flaskholder100ml_v4 (Autodesk Fusion 360 design; units mm, degrees)
Autodesk Fusion 360 part; units mm, degrees
sketch "Sketch1" plane through (0, 0, 0) normal (0, 0, 1) x (1, 0, 0)
  line L0 (99, 4.8) -> (99, -4.8)
  line L1 (-99, -4.8) -> (-99, 4.8)
  line L2 (-99, 9) -> (99, -9) construction
  line L3 (99, 9) -> (-99, -9) construction
  line L4 (6, 99) -> (-4.8, 99)
  line L5 (-4.8, -99) -> (4.8, -99)
  line L6 (9, 99) -> (-9, -99) construction
  line L7 (-9, 99) -> (9, -99) construction
  line L8 (-29, -9) -> (-94.8, -9)
  line L9 (94.8, -9) -> (29, -9)
  line L10 (0.8182, -9) -> (-0.8182, -9)
  line L11 (29, 9) -> (94.8, 9)
  line L12 (-94.8, 9) -> (-31.5, 9)
  line L13 (-0.8182, 9) -> (0.8182, 9)
  line L14 (-9, 94.8) -> (-9, 31.5)
  line L15 (-9, 0.8182) -> (-9, -0.8182)
  line L16 (-9, -29) -> (-9, -94.8)
  line L17 (9, -94.8) -> (9, -29)
  line L18 (9, 29) -> (9, 96)
  arc A0 (9, 29) -> (29, 9) centre (29, 29) ccw
  arc A1 (29, -9) -> (9, -29) centre (29, -29) ccw
  arc A2 (-9, -29) -> (-29, -9) centre (-29, -29) ccw
  arc A3 (-31.5, 9) -> (-9, 31.5) centre (-31.5, 31.5) ccw
  arc A4 (9, 96) -> (6, 99) centre (6, 96) ccw
  arc A5 (-4.8, 99) -> (-9, 94.8) centre (-4.8, 94.8) ccw
  arc A6 (-94.8, 9) -> (-99, 4.8) centre (-94.8, 4.8) ccw
  arc A7 (-99, -4.8) -> (-94.8, -9) centre (-94.8, -4.8) ccw
  arc A8 (99, 4.8) -> (94.8, 9) centre (94.8, 4.8) ccw
  arc A9 (94.8, -9) -> (99, -4.8) centre (94.8, -4.8) ccw
  arc A10 (-9, -94.8) -> (-4.8, -99) centre (-4.8, -94.8) ccw
  arc A11 (4.8, -99) -> (9, -94.8) centre (4.8, -94.8) ccw
  circle A12 centre (-86, 0) radius 1
  circle A13 centre (-31, 0) radius 1
  circle A14 centre (86, 0) radius 1
  circle A15 centre (31, 0) radius 1
  circle A16 centre (0, -86) radius 1
  circle A17 centre (0, -31) radius 1
  circle A18 centre (0, 86) radius 1
  circle A19 centre (0, 31) radius 1
  circle A20 centre (0, 0) radius 1
  dimension "d1" = 198
  dimension "d2" = 18
  dimension "d5" = 18
  dimension "d6" = 198
  dimension "d9" = 20
  dimension "d10" = 22.5
  dimension "d11" = 3
  dimension "d12" = 4.2
  dimension "d15" = 2
  dimension "d16" = 2
  dimension "d17" = 13
  dimension "d18" = 2
  dimension "d19" = 13
  dimension "d20" = 2
  dimension "d21" = 2
  dimension "d22" = 13
  dimension "d23" = 2
  dimension "d24" = 2
  dimension "d25" = 13
  dimension "d26" = 68
  dimension "d27" = 68
  dimension "d28" = 68
  dimension "d29" = 68
  dimension "d30" = 2
  constraint horizontal L12
  constraint perpendicular L0 L12
  constraint parallel L9 L12
  constraint parallel L0 L1
  constraint coincident L2 A20.centre
  constraint coincident L3 A20.centre
  constraint coincident A20.centre origin
  constraint horizontal L4
  constraint perpendicular L4 L14
  constraint parallel L4 L5
  constraint parallel L14 L17
  constraint coincident L6 A20.centre
  constraint coincident L7 A20.centre
  constraint coincident L6 L10.end
  constraint collinear L8 L9
  constraint coincident L7 L10.start
  constraint collinear L9 L10
  constraint coincident L6 L13.end
  constraint collinear L11 L12
  constraint coincident L7 L13.start
  constraint collinear L12 L13
  constraint coincident L2 L15.start
  constraint collinear L14 L15
  constraint coincident L3 L15.end
  constraint collinear L15 L16
  constraint collinear L17 L18
  constraint tangent L18 A0
  constraint tangent L11 A0
  constraint tangent L9 A1
  constraint tangent L17 A1
  constraint equal A0 A1
  constraint tangent L16 A2
  constraint tangent L8 A2
  constraint equal A0 A2
  constraint tangent L12 A3
  constraint tangent L14 A3
  constraint coincident L6.start L4
  constraint coincident L6.start L18
  constraint tangent L4 A4
  constraint tangent L18 A4
  constraint coincident L7.start L4
  constraint coincident L7.start L14
  constraint tangent L4 A5
  constraint tangent L14 A5
  constraint coincident L2.start L12
  constraint coincident L2.start L1
  constraint tangent L12 A6
  constraint tangent L1 A6
  constraint equal A5 A6
  constraint coincident L3.end L1
  constraint coincident L3.end L8
  constraint tangent L1 A7
  constraint tangent L8 A7
  constraint equal A5 A7
  constraint coincident L3.start L11
  constraint coincident L3.start L0
  constraint tangent L11 A8
  constraint tangent L0 A8
  constraint equal A5 A8
  constraint coincident L2.end L9
  constraint coincident L2.end L0
  constraint tangent L9 A9
  constraint tangent L0 A9
  constraint equal A5 A9
  constraint coincident L6.end L5
  constraint coincident L6.end L16
  constraint tangent L5 A10
  constraint tangent L16 A10
  constraint equal A5 A10
  constraint coincident L7.end L17
  constraint coincident L7.end L5
  constraint tangent L17 A11
  constraint tangent L5 A11
  constraint equal A5 A11
  constraint equal A12 A14
  measures "d1" distance of L2.end L3.end
  measures "d2" distance of L3.start L2.end
  measures "d5" distance of L6.end L7.end
  measures "d6" distance of L7.start L6.end
  measures "d9" radius of A0
  measures "d10" radius of A3
  measures "d11" radius of A4
  measures "d12" radius of A5
  measures "d15" diameter of A12
  measures "d16" diameter of A13
  measures "d17" distance of L1 A12.centre
  measures "d18" diameter of A15
  measures "d19" distance of L0 A14.centre
  measures "d20" diameter of A16
  measures "d21" diameter of A17
  measures "d22" distance of L5 A16.centre
  measures "d23" diameter of A18
  measures "d24" diameter of A19
  measures "d25" distance of L4 A18.centre
  measures "d26" distance of L4 A19.centre
  measures "d27" distance of L0 A15.centre
  measures "d28" distance of L1 A13.centre
  measures "d29" distance of L5 A17.centre
  measures "d30" diameter of A20
extrude "Extrude1" add sketch "Sketch1" along normal blind 3.175
equation "d1 = totalArmLenght"
equation "d2 = armWidth"
equation "totalArmLenght = 198 mm"
equation "armWidth = 18 mm"
equation "d5 = armWidth"
equation "d6 = totalArmLenght"
equation "tipBend = 13 mm"
equation "bottomBend = 68 mm"
equation "d17 = tipBend"
equation "d19 = tipBend"
equation "d22 = tipBend"
equation "d25 = tipBend"
equation "d26 = bottomBend"
equation "d27 = bottomBend"
equation "d28 = bottomBend"
equation "d29 = bottomBend"
